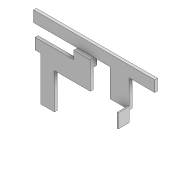
# Autodesk Inventor part: TerminalR
Saved by Autodesk Inventor 2021 (Build 250183000, 183)
## iProperties
Created: 2025-07-03
Part Number: TerminalR
Material: Generic
Document SubType Name: Modeling
Designer: Owner
Density: 1 g/cm^3
Appearance: Default
Author: Owner
Autodesk Inventor part; units mm, degrees
ref_plane "YZ Plane" through (0, 0, 0) normal (1, 0, 0) x (0, 1, 0)
ref_plane "XZ Plane" through (0, 0, 0) normal (0, 1, 0) x (-1, 0, 0)
ref_plane "XY Plane" through (0, 0, 0) normal (0, 0, 1) x (1, 0, 0)
sketch "Sketch1" plane through (0, 0, 0) normal (0, 0, 1) x (1, 0, 0)
  line L0 (11, -1) -> (11, 1)
  line L1 (11, 1) -> (-11, 1)
  line L2 (-11, 1) -> (-11, -1)
  line L3 (-11, -1) -> (11, 1) construction
  line L4 (11, -1) -> (-11, 1) construction
  line L5 (11, -1) -> (5.2, -1)
  line L6 (5.2, -1) -> (5.2, -8)
  line L7 (5.2, -8) -> (2.2, -8)
  line L8 (2.2, -8) -> (2.2, -1)
  line L9 (2.2, -1) -> (0, -1)
  line L10 (-10, -2.4556) -> (-3, -2.4556)
  line L11 (-3, -2.4556) -> (-3, -1)
  line L12 (-11, -1) -> (-3, -1)
  line L13 (0, -1) -> (2.2, -1)
  line L14 (5.2, -1) -> (11, -1)
  line L15 (-10, -2.4556) -> (-10, -4.4556)
  line L16 (-10, -4.4556) -> (-8.5, -4.4556)
  line L17 (-8.5, -4.4556) -> (-8.5, -12.4556)
  line L18 (-8.5, -12.4556) -> (-6.5, -12.4556)
  line L19 (-6.5, -12.4556) -> (-6.5, -4.4556)
  line L20 (-6.5, -4.4556) -> (0, -4.4556)
  line L21 (0, -1) -> (0, -4.4556)
  line L22 (5.2, -8) -> (5.7, -8)
  line L23 (5.7, -8) -> (5.7, -6)
  line L24 (5.7, -6) -> (5.2, -6)
  line L25 (5.2, -6) -> (5.2, -8)
  point P0 (0, 0)
  dimension "d0" = 22
  dimension "d1" = 2
  dimension "d2" = 5.8
  dimension "d3" = 7
  dimension "d4" = 3
  dimension "d5" = 2.2
  dimension "d8" = 7
  dimension "d9" = 2
  dimension "d11" = 8
  dimension "d12" = 2
  dimension "d13" = 0.5
  dimension "d14" = 2
  constraints: 52 end point, 16 perpendicular, 6 parallel, 4 horizontal, 2 midpoint, 2 point on line
  measures "d0" distance of L1.end L0.end
  measures "d1" distance of L0.end L0.start
  measures "d2" distance of L0.start L5.end
  measures "d3" distance of L5.end L6.end
  measures "d4" distance of L6.end L7.end
  measures "d5" distance of L8.end L9.end
  measures "d8" distance of L10.start L10.end
  measures "d9" distance of L10.start L15.end
  measures "d11" distance of L16.end L17.end
  measures "d12" distance of L17.end L18.end
  measures "d13" distance of L24.end L23.end
  measures "d14" distance of L23.end L22.end
extrude "Extrusion1" add sketch "Sketch1" along normal blind 0.5 contours L5 L6 L7 L8 L9 L21 L20 L19 L18 L17 L16 L15 L10 L11 L12 L2 L1 L0
sketch "Sketch2" plane through (0, 0, 0.5) normal (0, 0, 1) x (1, 0, 0)
  line L0 (5.2, -8) -> (5.2, -1) projected
  line L1 (5.2, -8) -> (5.7, -8)
  line L2 (5.7, -8) -> (5.7, -6)
  line L3 (5.7, -6) -> (5.2, -6)
  line L4 (5.2, -6) -> (5.2, -8)
  point P0 (0, 0)
  point P1 (5.2, -6)
  dimension "d17" = 0.5
  dimension "d18" = 2
  constraints: 8 end point, 2 parallel, 1 horizontal, 1 perpendicular
  measures "d17" distance of L3.end L2.end
  measures "d18" distance of L2.end L1.end
extrude "Extrusion2" add sketch "Sketch2" along normal blind 2
sketch "Sketch3" plane through (0, 0, 0.5) normal (0, 0, -1) x (-1, 0, 0)
  line L0 (-5.7, -6) -> (-5.2, -6) projected
  line L1 (-5.7, -8) -> (-5.7, -6) projected
  line L2 (-5.2, -8) -> (-5.7, -8) projected
  line L3 (-5.2, -8) -> (-5.2, -6) projected
  point P0 (0, 0)
extrude "Extrusion3" add sketch "Sketch3" along normal blind 0.5
sketch "Sketch4" plane through (0, 0, 0.5) normal (0, 0, 1) x (1, 0, 0)
  line L0 (11, 1) -> (-11, 1) projected
  line L1 (-11, 1) -> (-11, -1) projected
  line L2 (-11, -1) -> (-3, -1) projected
  line L3 (-3, -1) -> (-3, -2.4556) projected
  line L4 (-3, -2.4556) -> (-10, -2.4556) projected
  line L5 (-10, -2.4556) -> (-10, -4.4556) projected
  line L6 (-10, -4.4556) -> (-8.5, -4.4556) projected
  line L7 (-8.5, -4.4556) -> (-8.5, -12.4556) projected
  line L8 (-8.5, -12.4556) -> (-6.5, -12.4556) projected
  line L9 (-6.5, -12.4556) -> (-6.5, -4.4556) projected
  line L10 (-6.5, -4.4556) -> (0, -4.4556) projected
  line L11 (0, -4.4556) -> (0, -1) projected
  line L12 (0, -1) -> (2.2, -1) projected
  line L13 (2.2, -1) -> (2.2, -8) projected
  line L14 (2.2, -8) -> (5.2, -8) projected
  line L15 (5.2, -8) -> (5.2, -6) projected
  line L16 (5.2, -6) -> (5.2, -1) projected
  line L17 (5.2, -1) -> (11, -1) projected
  line L18 (11, -1) -> (11, 1) projected
  line L19 (-3, -1) -> (-3, -2.4556) projected
  line L20 (0, -1) -> (2.2, -1) projected
  line L21 (-3, -1) -> (0, -1)
  point P0 (0, 0)
  constraints: 2 end point, 1 collinear
extrude "Extrusion4" add sketch "Sketch4" along normal blind 0.7 contours L21 L11 L10 L9 L8 L7 L6 L5 L4 L3
sketch "Sketch5" plane through (0, 0, 0) normal (0, 0, -1) x (-1, 0, 0)
  line L0 (-11, 1) -> (11, 1) projected
  line L1 (-11, -1) -> (-11, 1) projected
  line L2 (-5.2, -1) -> (-11, -1) projected
  line L3 (-5.2, -6) -> (-5.2, -1) projected
  line L4 (-5.2, -6) -> (-5.7, -6) projected
  line L5 (-5.7, -6) -> (-5.7, -8) projected
  line L6 (-2.2, -8) -> (-5.7, -8) projected
  line L7 (-2.2, -1) -> (-2.2, -8) projected
  line L8 (0, -1) -> (-2.2, -1) projected
  line L9 (0, -4.4556) -> (0, -1) projected
  line L10 (6.5, -4.4556) -> (0, -4.4556) projected
  line L11 (6.5, -12.4556) -> (6.5, -4.4556) projected
  line L12 (8.5, -12.4556) -> (6.5, -12.4556) projected
  line L13 (8.5, -4.4556) -> (8.5, -12.4556) projected
  line L14 (10, -4.4556) -> (8.5, -4.4556) projected
  line L15 (10, -2.4556) -> (10, -4.4556) projected
  line L16 (3, -2.4556) -> (10, -2.4556) projected
  line L17 (3, -1) -> (3, -2.4556) projected
  line L18 (11, -1) -> (3, -1) projected
  line L19 (11, 1) -> (11, -1) projected
  line L20 (3, -2.4556) -> (0, -2.4556)
  line L21 (0, -4.4556) -> (0, -1) projected
  point P0 (0, 0)
  constraints: 2 end point, 1 perpendicular, 1 point on line
extrude "Extrusion5" cut sketch "Sketch5" against normal blind 0.5 contours L16 L15 L14 L13 L12 L11 L10 L9 L20
sketch "Sketch6" plane through (-6.5, -4.4556, 1.2) normal (0, -1, 0) x (1, 0, 0)
  line L0 (6.5, -0.7) -> (6.5, 0) projected
  line L1 (0, 0) -> (6.5, 0) projected
  line L2 (6.5, -0.7) -> (0, -0.7)
  line L3 (0, -0.7) -> (0, 0)
  line L4 (0, 0) -> (6.5, 0)
  line L5 (6.5, 0) -> (6.5, -0.7)
  point P0 (6.5, -1.2)
  constraints: 8 end point, 2 parallel, 1 horizontal, 1 perpendicular
extrude "Extrusion6" add sketch "Sketch6" along normal blind 1.5
sketch "Sketch7" plane through (5.7, -8, 2.5) normal (1, 0, 0) x (0, 0, -1)
  line L0 (0, 2) -> (2.5, 2) projected
  line L1 (0, 0) -> (0, 2) projected
  line L2 (2.5, 0) -> (0, 0) projected
  line L3 (2.5, 2) -> (2.5, 0) projected
  point P0 (2.5, 8)
extrude "Extrusion7" add sketch "Sketch7" along normal blind 0.5
sketch "Sketch8" plane through (5.2, -8, 0.5) normal (-1, 0, 0) x (0, 0, 1)
  line L0 (0, 0) -> (0, 2) projected
  line L1 (0, 0) -> (2, 0) projected
  line L2 (2, 2) -> (2, 0) projected
  line L3 (0, 2) -> (2, 2) projected
  point P0 (-0.5, 8)
extrude "Extrusion8" cut sketch "Sketch8" against normal blind 0.5
sketch "Sketch9" plane through (0, 0, 1.2) normal (0, 0, 1) x (1, 0, 0)
  line L0 (-10, -2.4556) -> (-10, -4.4556) projected
  line L1 (-10, -4.4556) -> (-8.5, -4.4556) projected
  line L2 (-8.5, -4.4556) -> (-8.5, -12.4556) projected
  line L3 (-8.5, -12.4556) -> (-6.5, -12.4556) projected
  line L4 (-6.5, -12.4556) -> (-6.5, -5.9556) projected
  line L5 (0, -5.9556) -> (-6.5, -5.9556) projected
  line L6 (0, -1) -> (0, -5.9556) projected
  line L7 (0, -1) -> (-3, -1) projected
  line L8 (-3, -1) -> (-3, -2.4556) projected
  line L9 (-3, -2.4556) -> (-10, -2.4556) projected
  point P0 (0, 0)
extrude "Extrusion9" cut sketch "Sketch9" against normal blind 0.2
sketch "Sketch10" plane through (0, 0, 0.5) normal (0, 0, -1) x (-1, 0, 0)
  line L0 (6.5, -12.4556) -> (6.5, -5.9556) projected
  line L1 (8.5, -12.4556) -> (6.5, -12.4556) projected
  line L2 (8.5, -4.4556) -> (8.5, -12.4556) projected
  line L3 (10, -4.4556) -> (8.5, -4.4556) projected
  line L4 (10, -2.4556) -> (10, -4.4556) projected
  line L5 (3, -2.4556) -> (10, -2.4556) projected
  line L6 (0, -2.4556) -> (3, -2.4556) projected
  line L7 (0, -5.9556) -> (0, -2.4556) projected
  line L8 (6.5, -5.9556) -> (0, -5.9556) projected
  point P0 (0, 0)
extrude "Extrusion10" add sketch "Sketch10" along normal blind 0.3
sketch "Sketch11" plane through (0, 0, 1) normal (0, 0, 1) x (1, 0, 0)
  line L0 (-3, -2.4556) -> (-3, -1) projected
  line L1 (-10, -2.4556) -> (-3, -2.4556) projected
  line L2 (-10, -4.4556) -> (-10, -2.4556) projected
  line L3 (-8.5, -4.4556) -> (-10, -4.4556) projected
  line L4 (-8.5, -12.4556) -> (-8.5, -4.4556) projected
  line L5 (-6.5, -12.4556) -> (-8.5, -12.4556) projected
  line L6 (-6.5, -5.9556) -> (-6.5, -12.4556) projected
  line L7 (0, -5.9556) -> (-6.5, -5.9556) projected
  line L8 (0, -1) -> (0, -5.9556) projected
  line L9 (-3, -1) -> (0, -1) projected
  point P0 (0, 0)
extrude "Extrusion11" cut sketch "Sketch11" against normal blind 0.3
sketch "Sketch12" plane through (0, 0, 0.7) normal (0, 0, 1) x (1, 0, 0)
  line L0 (-10, -4.4556) -> (-10, -2.4556) projected
  line L1 (-8.5, -4.4556) -> (-10, -4.4556) projected
  line L2 (-8.5, -12.4556) -> (-8.5, -4.4556) projected
  line L3 (-6.5, -12.4556) -> (-8.5, -12.4556) projected
  line L4 (-6.5, -5.9556) -> (-6.5, -12.4556) projected
  line L5 (0, -5.9556) -> (-6.5, -5.9556) projected
  line L6 (0, -1) -> (0, -5.9556) projected
  line L7 (-3, -1) -> (0, -1) projected
  line L8 (-3, -2.4556) -> (-3, -1) projected
  line L9 (-10, -2.4556) -> (-3, -2.4556) projected
  point P0 (0, 0)
extrude "Extrusion12" add sketch "Sketch12" along normal blind 0.5
sketch "Sketch13" plane through (0, 0, 0.2) normal (0, 0, -1) x (-1, 0, 0)
  line L0 (8.5, -12.4556) -> (8.5, -4.4556) projected
  line L1 (8.5, -4.4556) -> (10, -4.4556) projected
  line L2 (10, -4.4556) -> (10, -2.4556) projected
  line L3 (10, -2.4556) -> (3, -2.4556) projected
  line L4 (0, -2.4556) -> (3, -2.4556) projected
  line L5 (0, -2.4556) -> (0, -5.9556) projected
  line L6 (0, -5.9556) -> (6.5, -5.9556) projected
  line L7 (6.5, -5.9556) -> (6.5, -12.4556) projected
  line L8 (6.5, -12.4556) -> (8.5, -12.4556) projected
  point P0 (0, 0)
extrude "Extrusion13" cut sketch "Sketch13" against normal blind 0.5
sketch "Sketch14" plane through (6.2, -8, 2.5) normal (1, 0, 0) x (0, 0, -1)
  line L0 (0, 0) -> (2.5, 0) projected
  line L1 (2.5, 0) -> (2.5, 2) projected
  line L2 (2.5, 2) -> (0, 2) projected
  line L3 (0, 2) -> (0, 0) projected
  point P0 (2.5, 8)
extrude "Extrusion14" add sketch "Sketch14" along normal blind 0.3
sketch "Sketch15" plane through (5.7, -8, 0.5) normal (-1, 0, 0) x (0, 0, 1)
  line L0 (2, 2) -> (2, 0) projected
  line L1 (0, 2) -> (2, 2) projected
  line L2 (0, 0) -> (0, 2) projected
  line L3 (2, 0) -> (0, 0) projected
  point P0 (-0.5, 8)
extrude "Extrusion15" cut sketch "Sketch15" against normal blind 0.3
sketch "Sketch16" plane through (2.2, -8, 0) normal (-1, 0, 0) x (0, 0, 1)
  line L0 (0, 7) -> (0, 0) projected
  line L1 (0, 0) -> (0.5, 0) projected
  line L2 (0.5, 7) -> (0.5, 0) projected
  line L3 (0, 7) -> (0.5, 7) projected
  point P0 (0, 8)
extrude "Extrusion16" add sketch "Sketch16" along normal blind 0.04
sketch "Sketch17" plane through (6, -8, 0.5) normal (-1, 0, 0) x (0, 0, 1)
  line L0 (0, 0) -> (0, 2) projected
  line L1 (2, 0) -> (0, 0) projected
  line L2 (2, 2) -> (2, 0) projected
  line L3 (0, 2) -> (2, 2) projected
  point P0 (-0.5, 8)
extrude "Extrusion17" add sketch "Sketch17" along normal blind 0.125
sketch "Sketch18" plane through (6.5, -8, 2.5) normal (1, 0, 0) x (0, 0, -1)
  line L0 (2.5, 0) -> (2.5, 2) projected
  line L1 (2.5, 2) -> (0, 2) projected
  line L2 (0, 2) -> (0, 0) projected
  line L3 (0, 0) -> (2.5, 0) projected
  point P0 (2.5, 8)
extrude "Extrusion18" cut sketch "Sketch18" against normal blind 0.125
sketch "Sketch19" plane through (5.2, -1, 0.5) normal (1, 0, 0) x (0, 0, -1)
  line L0 (0, -5) -> (0.5, -5) projected
  line L1 (0.5, -5) -> (0.5, 0) projected
  line L2 (0.5, 0) -> (0, 0) projected
  line L3 (0, -5) -> (0, 0) projected
  point P0 (0.5, 1)
extrude "Extrusion19" add sketch "Sketch19" along normal blind 1.175
sketch "Sketch20" plane through (5.875, -6, 2.5) normal (0, 1, 0) x (1, 0, 0)
  line L0 (0.5, 2) -> (0, 2) projected
  line L1 (0, 0) -> (0, 2) projected
  line L2 (0, 0) -> (0.5, 0) projected
  line L3 (0.5, 0) -> (0.5, 2) projected
  point P0 (-5.875, 2.5)
extrude "Extrusion20" add sketch "Sketch20" along normal blind 2
sketch "Sketch21" plane through (2.16, -8, 0) normal (0, -1, 0) x (1, 0, 0)
  line L0 (4.215, 0) -> (4.215, 2.5) projected
  line L1 (3.715, 2.5) -> (4.215, 2.5) projected
  line L2 (3.715, 0.5) -> (3.715, 2.5) projected
  line L3 (3.715, 0.5) -> (0, 0.5) projected
  line L4 (0, 0) -> (0, 0.5) projected
  line L5 (4.215, 0) -> (0, 0) projected
  point P0 (-2.16, 0)
extrude "Extrusion21" cut sketch "Sketch21" against normal blind 1.96
sketch "Sketch22" plane through (5.875, -4, 2.5) normal (0, 1, 0) x (1, 0, 0)
  line L0 (0.5, 0) -> (0.5, 2) projected
  line L1 (0, 2) -> (0.5, 2) projected
  line L2 (0, 2) -> (0, 0) projected
  line L3 (0, 0) -> (0.5, 0) projected
  point P0 (-5.875, 2.5)
extrude "Extrusion22" cut sketch "Sketch22" against normal blind 1.5
sketch "Sketch23" plane through (2.16, -6.04, 0) normal (0, -1, 0) x (1, 0, 0)
  line L0 (0, 0.5) -> (3.715, 0.5) projected
  line L1 (4.215, 2.5) -> (4.215, 0) projected
  line L2 (3.715, 0.5) -> (4.215, 0.5)
  line L3 (4.215, 0.5) -> (4.215, 2.5)
  line L4 (4.215, 2.5) -> (3.715, 2.5)
  line L5 (3.715, 2.5) -> (3.715, 0.5)
  point P0 (-2.16, 0)
  constraints: 8 end point, 2 parallel, 1 horizontal, 1 perpendicular
extrude "Extrusion23" add sketch "Sketch23" along normal blind 2
sketch "Sketch24" plane through (2.16, -8, 0) normal (-1, 0, 0) x (0, 0, 1)
  line L0 (0, 1.96) -> (0.5, 1.96) projected
  line L1 (0.5, 1.96) -> (0.5, 7) projected
  line L2 (0, 7) -> (0.5, 7) projected
  line L3 (0, 7) -> (0, 1.96) projected
  point P0 (0, 8)
extrude "Extrusion24" cut sketch "Sketch24" against normal blind 0.75
sketch "Sketch25" plane through (5.875, -8, 0.5) normal (-1, 0, 0) x (0, 0, 1)
  line L0 (2, 2.5) -> (0, 2.5) projected
  line L1 (0, 1.96) -> (0, 2.5) projected
  line L2 (0, 1.96) -> (0, -0.04) projected
  line L3 (2, -0.04) -> (0, -0.04) projected
  line L4 (2, -0.04) -> (2, 2.5) projected
  point P0 (-0.5, 8)
extrude "Extrusion25" cut sketch "Sketch25" against normal blind 0.3
sketch "Sketch26" plane through (-8.5, -12.4556, 1.2) normal (-1, 0, 0) x (0, 0, 1)
  line L0 (-0.5, 8) -> (-0.5, 0) projected
  line L1 (-0.5, 0) -> (0, 0) projected
  line L2 (0, 8) -> (0, 0) projected
  line L3 (-0.5, 8) -> (0, 8) projected
  point P0 (-1.2, 12.4556)
extrude "Extrusion26" add sketch "Sketch26" along normal blind 0.5
body "Solid1"
